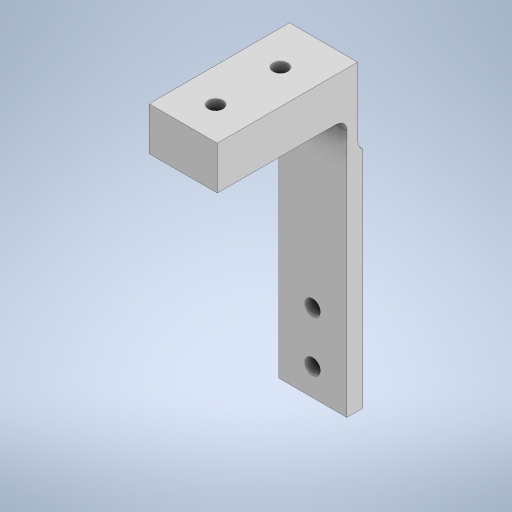
# Autodesk Inventor part: Tensioner Mount V1
Saved by Autodesk Inventor 2024.2 (Build 282272000, 272)
## iProperties
Created: 2024-08-08
Part Number: Tensioner Mount V1
Material: Generic
Document SubType Name: Modeling
Designer: balmo
Density: 1 g/cm^3
Appearance: Default
Author: balmo
## iProperties of the stored document Tensioner Mount V1_3DPrint.ipt
Created: 2024-08-09
Part Number: Tensioner Mount V1_3DPrint
Material: Generic
Document SubType Name: Modeling
Designer: balmo
Density: 1 g/cm^3
Appearance: Default
Author: balmo
Autodesk Inventor part; units mm, degrees
ref_plane "YZ Plane" through (0, 0, 0) normal (1, 0, 0) x (0, 1, 0)
ref_plane "XZ Plane" through (0, 0, 0) normal (0, 1, 0) x (-1, 0, 0)
ref_plane "XY Plane" through (0, 0, 0) normal (0, 0, 1) x (1, 0, 0)
sketch "Sketch1" plane through (0, 0, 0) normal (0, 0, 1) x (1, 0, 0)
  line L0 (0, 0) -> (20.066, 0)
  line L1 (20.066, 0) -> (20.066, 88.9)
  line L2 (20.066, 88.9) -> (0, 88.9)
  line L3 (0, 88.9) -> (0, 0)
  circle A0 centre (10.033, 8) radius 2.25
  circle A1 centre (10.033, 23) radius 2.25
  dimension "d0" = 20.066
  dimension "d1" = 88.9
  dimension "d10" = 8
  dimension "d11" = 15
  dimension "d12" = 4.5
  dimension "d13" = 4.5
  constraints: 8 end point, 2 centre point, 2 parallel, 1 horizontal, 1 perpendicular
  measures "d0" distance of L2.end L1.end
  measures "d1" distance of L2.end L0.start
  measures "d10" distance from line of L0 A0.centre
  measures "d11" distance of A1.centre A0.centre
  measures "d12" diameter of A0
  measures "d13" diameter of A1
extrude "Extrusion1" add sketch "Sketch1" along normal blind 3.175
sketch "Sketch2" plane through (0, 0, 3.175) normal (0, 0, 1) x (1, 0, 0)
  line L0 (0, 88.9) -> (0, 0) projected
  line L1 (20.066, 0) -> (20.066, 88.9) projected
  line L2 (0, 88.9) -> (20.066, 88.9)
  line L3 (20.066, 88.9) -> (20.066, 76.2)
  line L4 (20.066, 76.2) -> (0, 76.2)
  line L5 (0, 76.2) -> (0, 88.9)
  point P0 (0, 76.2)
  dimension "d4" = 12.7
  constraints: 8 end point, 2 parallel, 1 horizontal, 1 perpendicular, 1 point on line
  measures "d4" distance of L2.end L3.end
extrude "Extrusion2" add sketch "Sketch2" along normal blind 38.1
sketch "Sketch3" plane through (0, 0, 0) normal (0, 0, -1) x (-1, 0, 0)
  line L0 (-20.066, 0) -> (-20.066, 88.9) projected
  line L1 (0, 0) -> (-20.066, 0) projected
  line L2 (0, 88.9) -> (0, 0) projected
  line L3 (-20.066, 88.9) -> (0, 88.9) projected
  line L4 (-20.066, 66.04) -> (0, 66.04)
  line L5 (0, 66.04) -> (0, 0)
  line L6 (0, 0) -> (-20.066, 0)
  line L7 (-20.066, 0) -> (-20.066, 66.04)
  point P0 (0, 66.04)
  dimension "d7" = 22.86
  constraints: 8 end point, 2 parallel, 1 horizontal, 1 perpendicular, 1 point on line
  measures "d7" distance between parallel lines of L4 L3
extrude "Extrusion3" add sketch "Sketch3" along normal blind 1.524 contours L0 L4 L2 L1
sketch "Sketch4" plane through (10.033, 23, 0) normal (0, 0, 1) x (1, 0, 0)
  circle A0 centre (0, -15) radius 2.25 projected
  circle A1 centre (0, 0) radius 2.25 projected
  point P0 (-10.033, -23)
extrude "Extrusion4" cut sketch "Sketch4" against normal blind 3.175
sketch "Sketch5" plane through (0, 76.2, 3.175) normal (0, -1, 0) x (1, 0, 0)
  line L0 (20.066, 0) -> (0, 0) projected
  line L1 (20.066, 0) -> (20.066, 38.1) projected
  line L2 (0, 38.1) -> (20.066, 38.1) projected
  line L3 (0, 0) -> (0, 38.1) projected
  circle A0 centre (10.033, 28.575) radius 2.159
  circle A1 centre (10.033, 9.525) radius 2.159
  point P0 (0, -3.175)
  point P1 (10.033, 38.1)
  dimension "d16" = 4.318
  dimension "d17" = 4.318
  dimension "d18" = 9.525
  dimension "d19" = 9.525
  constraints: 2 centre point, 1 midpoint
  measures "d16" diameter of A0
  measures "d17" diameter of A1
  measures "d18" distance of point (10.033, 38.1) A0.centre
  measures "d19" distance from line of L0 A1.centre
extrude "Extrusion5" cut sketch "Sketch5" against normal through all contours A0 | A1
fillet "Fillet1" radius 3.175 1 edges at (10.033, 76.2, 3.175)
chamfer "Chamfer1" distance 2.286 angle 45 2 edges at (7.874, 76.2, 31.75) (7.874, 76.2, 12.7)
fillet "Fillet2" radius 3.175 1 edges at (10.033, 66.04, 0)
body "Solid1"
